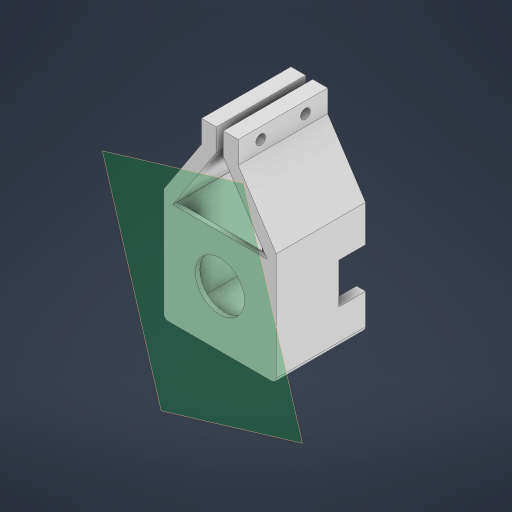
# Autodesk Inventor part: nema_brackets_and_lineguides
Saved by Autodesk Inventor 2024 (Build 280153000, 153)
## iProperties
Created: 2026-03-24
Part Number: nema_brackets_and_lineguides
Material: PET Plastic
Document SubType Name: Modeling
Designer: schar
Density: 1.541 g/cm^3
Appearance: Polycarbonate - Clear
Mass: 63.5811 g
Surface Area: 205.52 cm^2
Volume: 41.2597 cm^3
Author: schar
Autodesk Inventor part; units mm, degrees
ref_plane "YZ Plane" through (0, 0, 0) normal (1, 0, 0) x (0, 1, 0)
ref_plane "XZ Plane" through (0, 0, 0) normal (0, 1, 0) x (-1, 0, 0)
ref_plane "XY Plane" through (0, 0, 0) normal (0, 0, 1) x (1, 0, 0)
sketch "Sketch1" plane through (0, 0, 0) normal (0, 0, 1) x (1, 0, 0)
  line L0 (21.15, 2.975) -> (-21.15, 2.975)
  line L1 (-21.15, 2.975) -> (-21.15, -39.325)
  line L2 (-21.15, -39.325) -> (21.15, -39.325)
  line L3 (21.15, -39.325) -> (21.15, 2.975)
  line L4 (21.15, 2.975) -> (-21.15, -39.325) construction
  line L5 (-21.15, 2.975) -> (21.15, -39.325) construction
  line L6 (-25.15, 6.975) -> (25.15, 6.975)
  line L7 (25.15, 6.975) -> (25.15, -43.325)
  line L8 (25.15, -43.325) -> (-25.15, -43.325)
  line L9 (-25.15, -43.325) -> (-25.15, 6.975)
  line L10 (-25.15, 6.975) -> (25.15, -43.325) construction
  line L11 (25.15, 6.975) -> (-25.15, -43.325) construction
  line L12 (20.4961, 3.8233) -> (1.5, 32.825) projected
  line L13 (-1.5, 32.825) -> (-20.4961, 3.8233) projected
  line L14 (1.5, 32.825) -> (18.4317, 6.975)
  line L15 (-18.4317, 6.975) -> (-1.5, 32.825)
  line L16 (-25.15, 6.975) -> (-8.2183, 32.825)
  line L17 (0, 11.6716) -> (0, 114.7997)
  line L18 (25.15, 6.975) -> (8.2182, 32.825)
  line L19 (1.5, 32.825) -> (1.5, 42.825)
  line L20 (8.2182, 32.825) -> (8.2182, 42.825)
  line L21 (8.2182, 42.825) -> (1.5, 42.825)
  line L22 (-8.2183, 32.825) -> (-8.2183, 42.825)
  line L23 (-1.5, 32.825) -> (-1.5, 42.825)
  line L24 (-1.5, 42.825) -> (-8.2183, 42.825)
  line L25 (21.15, 2.975) -> (21.15, 6.975)
  line L26 (-21.15, 2.975) -> (-21.15, 6.975)
  line L27 (20.4961, 3.8233) -> (22.5003, 0.7634)
  line L28 (21.0517, 2.975) -> (21.15, 2.975)
  line L29 (-20.4961, 3.8233) -> (-22.8629, 0.2099)
  point P0 (0, 0)
  point P1 (0, -18.175)
  point P2 (-21.0517, 2.975)
  dimension "d0" = 42.3
  dimension "d1" = 42.3
  dimension "d2" = 50.3
  dimension "d3" = 50.3
  dimension "d4" = 10
  constraints: 56 end point, 10 point on line, 6 perpendicular, 5 parallel, 4 midpoint, 4 vertical, 3 collinear, 2 coincident, 2 horizontal, 1 symmetric about line, 3 other
  measures "d0" distance of L2.end L1.end
  measures "d1" distance of L1.end L0.end
  measures "d2" distance of L7.end L8.end
  measures "d3" distance of L6.end L7.end
  measures "d4" distance of L14.start L19.end
extrude "Extrusion1" add sketch "Sketch1" against normal blind 40 contours L25 L6 L7 L8 L9 L26 L1 L2 L3 | L0 L27 L12 L6 L25 | L6 L12 L19 L21 L20 L18 | L0 L26 L6 L13 L29 | L6 L16 L22 L24 L23 L13
sketch "Sketch2" plane through (25.15, -43.325, 0) normal (1, 0, 0) x (0, 0, -1)
  line L0 (30, 31.85) -> (31.6, 31.85)
  line L1 (30, 28.85) -> (30, 31.85)
  line L2 (30, 17.85) -> (30, 20.85)
  line L3 (31.6, 17.85) -> (30, 17.85)
  line L4 (39, 16.95) -> (36.4, 16.95)
  line L5 (39.4, 16.95) -> (39.4, 32.75)
  line L6 (39, 33.15) -> (36.4, 33.15)
  line L7 (31.6, 17.85) -> (31.6, 31.85)
  line L8 (31.6, 24.85) -> (40, 24.85)
  line L9 (40, 46.3) -> (40, 4)
  line L10 (40, 24.85) -> (40, 33.85)
  line L11 (40, 33.85) -> (28, 33.85)
  line L12 (28, 33.85) -> (28, 15.85)
  line L13 (28, 15.85) -> (40, 15.85)
  line L14 (40, 15.85) -> (40, 33.85)
  point P0 (0, 43.325)
  point P1 (40, 15.85)
extrude "Extrusion2" cut sketch "Sketch2" against normal up to surface (4 mm away)
ref_plane "Work Plane1" through (0, -18.475, 8) normal (0, 0, -1) x (0.9576506, 0.287933, 0)
fillet "Fillet1" radius 2 2 edges at (25.15, -43.325, -20) (-25.15, -43.325, -20)
sketch "Sketch20" plane through (8.2182, 32.825, 0) normal (1, 0, 0) x (0, 0, -1)
  line L0 (0, 0) -> (40, 0) projected
  line L1 (40, 0) -> (30, 0)
  line L2 (30, 0) -> (30, 5)
  line L3 (0, 10) -> (40, 10) projected
  line L4 (30, 5) -> (10, 5)
  circle A0 centre (30, 5) radius 2.15
  circle A1 centre (10, 5) radius 2.15
  point P0 (0, -32.825)
  dimension "d85" = 10
  dimension "d86" = 5
  dimension "d87" = 20
  dimension "d88" = 4.3
  dimension "d89" = 4.3
  constraints: 6 end point, 2 centre point, 2 coincident, 1 horizontal, 1 perpendicular, 1 point on line
  measures "d85" distance of L0.end L1.end
  measures "d86" distance of L1.end L2.end
  measures "d87" distance of L2.end L4.end
  measures "d88" diameter of A0
  measures "d89" diameter of A1
extrude "Extrusion18" cut sketch "Sketch20" against normal through all
sketch "Sketch21" plane through (0, 0, 0) normal (0, 0, 1) x (1, 0, 0)
  line L0 (-21.15, -39.325) -> (-21.15, 2.975) projected
  line L1 (21.15, -39.325) -> (-21.15, -39.325) projected
  line L2 (-21.15, 2.975) -> (21.15, 2.975)
  line L3 (21.15, 2.975) -> (21.15, -39.325)
  line L4 (21.15, -39.325) -> (-21.15, -39.325)
  line L5 (-21.15, -39.325) -> (-21.15, 2.975)
  line L6 (21.15, -39.325) -> (0, -39.325)
  line L7 (0, -39.325) -> (0, -18.175)
  line L8 (0, -18.175) -> (21.15, -18.175)
  line L9 (21.15, -18.175) -> (21.15, -39.325)
  circle A0 centre (0, -18.175) radius 11
  point P0 (0, 0)
  dimension "d92" = 22
  constraints: 16 end point, 4 parallel, 2 horizontal, 2 perpendicular, 1 centre point, 1 coincident
  measures "d92" diameter of A0
extrude "Extrusion19" add sketch "Sketch21" against normal blind 2 contours L0 L2 L3 L8 A0 L7 L1 | L7 A0 L8 L3 L1
body "Solid1"
